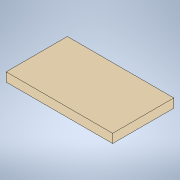
# Autodesk Inventor part: HalterungMotorregler
Saved by Autodesk Inventor 2020.3 (Build 243373010, 373A)
## iProperties
Created: 2021-02-05
Part Number: HalterungMotorregler
Material: Generisch
Document SubType Name: Modeling
Designer: Stefan
Density: 1 g/cm^3
Appearance: Pappel
Author: Stefan
Autodesk Inventor part; units mm, degrees
ref_plane "YZ Plane" through (0, 0, 0) normal (1, 0, 0) x (0, 1, 0)
ref_plane "XZ Plane" through (0, 0, 0) normal (0, 1, 0) x (-1, 0, 0)
ref_plane "XY Plane" through (0, 0, 0) normal (0, 0, 1) x (1, 0, 0)
sketch "Skizze1" plane through (0, 0, 0) normal (0, 1, 0) x (-1, 0, 0)
  line L0 (32.7365, 12.4043) -> (-87.2635, 12.4043)
  line L1 (-87.2635, 12.4043) -> (-87.2635, -56.5957)
  line L2 (-87.2635, -56.5957) -> (32.7365, -56.5957)
  line L3 (32.7365, -56.5957) -> (32.7365, 12.4043)
  point P0 (0, 0)
  dimension "d0" = 120
  dimension "d1" = 69
  constraints: 8 end point, 2 parallel, 1 horizontal, 1 perpendicular
  measures "d0" distance of L2.end L1.end
  measures "d1" distance of L1.end L0.end
extrude "Extrusion1" add sketch "Skizze1" along normal blind 10
